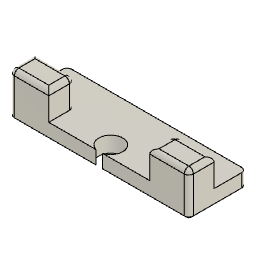
Handlebar Spacer (Autodesk Fusion 360 design; units mm, degrees)
Autodesk Fusion 360 part; units mm, degrees
sketch "Sketch1" plane through (0, 0, 0) normal (0, 0, 1) x (1, 0, 0)
  line L0 (19.5, 10) -> (-19.5, 10)
  line L1 (-19.5, 10) -> (-19.5, -10)
  line L2 (-19.5, -10) -> (19.5, -10)
  line L3 (19.5, -10) -> (19.5, 10)
  line L4 (19.5, 10) -> (-19.5, -10) construction
  line L5 (-19.5, 10) -> (19.5, -10) construction
  circle A0 centre (0, 0) radius 2.6
  dimension "d1" = 5.2
  dimension "d2" = 39
  dimension "d3" = 20
  constraint horizontal L0
  constraint perpendicular L0 L1
  constraint parallel L0 L2
  constraint parallel L1 L3
  constraint coincident L4 A0.centre
  constraint coincident L5 A0.centre
  constraint coincident A0.centre origin
  measures "d1" diameter of A0
  measures "d2" distance of L0.start L0.end
  measures "d3" distance of L0.start L2.end
extrude "Extrude1" add sketch "Sketch1" along normal blind 3.4
sketch "Sketch2" plane through (0, 0, 3.4) normal (0, 0, 1) x (-1, 0, 0)
  circle A0 centre (0, 0) radius 2.6
  line L0 (-19.5, 10) -> (-19.5, -10)
  line L1 (-19.5, -10) -> (19.5, -10)
  line L2 (19.5, -10) -> (19.5, 10)
  line L3 (19.5, 10) -> (-19.5, 10)
  line L4 (19.5, 3) -> (-19.5, 3)
  line L5 (19.5, -3) -> (-19.5, -3)
  line L6 (-19.5, 3) -> (19.5, -3) construction
  dimension "d7" = 6
  constraint coincident L2 L4.start
  constraint coincident L0 L4.end
  constraint perpendicular L0 L4
  constraint coincident L2 L5.start
  constraint coincident L0 L5.end
  constraint perpendicular L0 L5
  constraint coincident A0.centre L6
  measures "d7" distance of L4 L5
extrude "Extrude2" add sketch "Sketch2" along normal blind 6 contours L0 L2 L4 L5
extrude "Extrude5" cut 1 faces at (-6.5, -10, 2.2667) along direction (0, 1, 0) up to surface (7 mm away)
sketch "Sketch3" plane through (0, 0, 9.4) normal (0, 0, 1) x (-1, 0, 0)
  line L0 (19.5, 3) -> (-19.5, 3)
  line L1 (-19.5, 3) -> (-19.5, -3)
  line L2 (-19.5, -3) -> (19.5, -3)
  line L3 (19.5, -3) -> (19.5, 3)
  line L4 (11, -3) -> (11, 3)
  line L5 (-11, -3) -> (-11, 3)
  circle A0 centre (0, 0) radius 2.6
  dimension "d11" = 11
  dimension "d12" = 11
  constraint coincident L2 L4.start
  constraint coincident L0 L4.end
  constraint perpendicular L0 L4
  constraint coincident L2 L5.start
  constraint coincident L0 L5.end
  constraint perpendicular L0 L5
  measures "d11" distance of A0.centre L4
  measures "d12" distance of A0.centre L5
extrude "Extrude3" cut sketch "Sketch3" against normal up to surface (6 mm away) contours L0 L2 L4 L5
extrude "Extrude4" cut 1 faces at (-16.6667, -3, 4.2667) along direction (0, 1, 0) blind 0.5
fillet "Fillet2" radius 1 6 edges at (-19.5, 10, 1.7) (-19.5, -2.5, 4.7) (19.5, 10, 1.7) (19.5, -2.5, 4.7) (11, 3, 6.4) (-11, 3, 6.4)
fillet "Fillet1" radius 1 8 edges at (-15.25, -2.5, 9.4) (-19.5, 0.25, 9.4) (-11, 0.25, 9.4) (-15.25, 3, 9.4) (11, 0.25, 9.4) (15.25, -2.5, 9.4) (15.25, 3, 9.4) (19.5, 0.25, 9.4)
chamfer "Chamfer1" distance 0.5 angle 45 3 edges at (-19.5, 3.75, 0) (0, 10, 0) (19.5, 3.75, 0)
